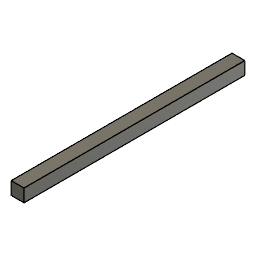
Beam_360mm (Autodesk Fusion 360 design; units mm, degrees)
part number: 2026-09-01-21-14-56-900
Autodesk Fusion 360 part; units mm, degrees
sketch "Sketch1" plane through (0, 0, 0) normal (0, 0, 1) x (1, 0, 0)
  line L0 (-10.5, -10.5) -> (10.5, -10.5)
  line L1 (10.5, -10.5) -> (10.5, 10.5)
  line L2 (10.5, 10.5) -> (-10.5, 10.5)
  line L3 (-10.5, 10.5) -> (-10.5, -10.5)
extrude "Extrude1" add sketch "Sketch1" along normal blind 360
named bodies: "Beam_360mm"
